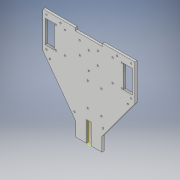
# Autodesk Inventor part: Very real base
Saved by Autodesk Inventor 2019 (Build 230136000, 136)
## iProperties
Created: 2018-08-20
Part Number: Very real base
Material: Generic
Document SubType Name: Modeling
Designer: kalakuntla1297
Density: 1 g/cm^3
Appearance: Default
Author: kalakuntla1297
Autodesk Inventor part; units mm, degrees
ref_plane "YZ Plane" through (0, 0, 0) normal (1, 0, 0) x (0, 1, 0)
ref_plane "XZ Plane" through (0, 0, 0) normal (0, 1, 0) x (-1, 0, 0)
ref_plane "XY Plane" through (0, 0, 0) normal (0, 0, 1) x (1, 0, 0)
sketch "Sketch1" plane through (0, 0, 0) normal (0, 0, 1) x (1, 0, 0)
  line L0 (0, 0) -> (508, 0)
  line L1 (508, 0) -> (508, -185.42)
  line L2 (0, 0) -> (0, -185.42)
  line L3 (254, 0) -> (254, -508)
  line L4 (254, -508) -> (266.7, -508)
  line L5 (254, -508) -> (241.3, -508)
  line L6 (266.7, -508) -> (266.7, -393.7)
  line L7 (241.3, -508) -> (241.3, -393.7)
  line L8 (266.7, -508) -> (326.39, -508)
  line L9 (241.3, -508) -> (181.61, -508)
  line L10 (326.39, -508) -> (326.39, -431.8)
  line L11 (326.39, -431.8) -> (508, -185.42)
  line L12 (241.3, -393.7) -> (266.7, -393.7)
  line L13 (12.7, -22.1996) -> (63.5, -22.1996)
  line L14 (63.5, -22.1996) -> (63.5, -149.1996)
  line L15 (63.5, -149.1996) -> (12.7, -149.1996)
  line L16 (12.7, -149.1996) -> (12.7, -22.1996)
  line L17 (495.3, -22.1996) -> (444.5, -22.1996)
  line L18 (444.5, -22.1996) -> (444.5, -149.1996)
  line L19 (444.5, -149.1996) -> (495.3, -149.1996)
  line L20 (495.3, -149.1996) -> (495.3, -22.1996)
  circle A0 centre (71.374, -24.13) radius 4.064
  circle A1 centre (122.174, -24.13) radius 4.064
  circle A2 centre (71.374, -147.2692) radius 4.064
  circle A3 centre (122.174, -147.2692) radius 4.064
  circle A4 centre (385.826, -147.2692) radius 4.064
  circle A5 centre (436.626, -147.2692) radius 4.064
  circle A6 centre (436.626, -24.13) radius 4.064
  circle A7 centre (385.826, -24.13) radius 4.064
  line L21 (0, -185.42) -> (508, -185.42)
  line L22 (181.61, -508) -> (181.61, -431.8)
  line L23 (181.61, -431.8) -> (0, -185.42)
  dimension "d0" = 508
  dimension "d1" = 185.42
  dimension "d2" = 185.42
  dimension "d3" = 508
  dimension "d4" = 12.7
  dimension "d5" = 12.7
  dimension "d6" = 114.3
  dimension "d7" = 59.69
  dimension "d8" = 59.69
  dimension "d9" = 76.2
  dimension "d10" = 22.1996
  dimension "d11" = 22.1996
  dimension "d12" = 12.7
  dimension "d13" = 12.7
  dimension "d14" = 50.8
  dimension "d15" = 50.8
  dimension "d16" = 149.1996
  dimension "d17" = 149.1996
  dimension "d18" = 8.128
  dimension "d19" = 8.128
  dimension "d20" = 8.128
  dimension "d21" = 8.128
  dimension "d22" = 24.13
  dimension "d23" = 24.13
  dimension "d24" = 147.2692
  dimension "d25" = 147.2692
  dimension "d26" = 7.874
  dimension "d27" = 58.674
  dimension "d28" = 7.874
  dimension "d29" = 58.674
  constraints: 48 end point, 8 centre point, 7 horizontal, 7 vertical, 4 parallel, 4 symmetric about line, 3 perpendicular, 1 midpoint, 1 point on line, 4 other
  measures "d0" distance of L0.start L1.start
  measures "d1" distance of L1.start L11.end
  measures "d2" distance of L0.start L21.start
  measures "d3" distance of L3.start L3.end
  measures "d4" distance of L3.end L6.start
  measures "d5" distance of L3.end L9.start
  measures "d6" distance of L6.start L12.end
  measures "d7" distance of L6.start L10.start
  measures "d8" distance of L9.start L9.end
  measures "d9" distance of L10.start L11.start
  measures "d10" distance between parallel lines of L0 L13
  measures "d11" distance between parallel lines of L0 L17
  measures "d12" distance between parallel lines of L2 L16
  measures "d13" distance between parallel lines of L1 L20
  measures "d14" distance of L14.end L16.start
  measures "d15" distance of L18.end L19.end
  measures "d16" distance between parallel lines of L0 L19
  measures "d17" distance between parallel lines of L0 L15
  measures "d18" diameter of A1
  measures "d19" diameter of A3
  measures "d20" diameter of A2
  measures "d21" diameter of A0
  measures "d22" distance from line of L0 A0.centre
  measures "d23" distance from line of L0 A1.centre
  measures "d24" distance from line of L0 A2.centre
  measures "d25" distance from line of L0 A3.centre
  measures "d26" distance from line of L14 A0.centre
  measures "d27" distance from line of L14 A1.centre
  measures "d28" distance from line of L14 A2.centre
  measures "d29" distance from line of L14 A3.centre
extrude "Extrusion1" add sketch "Sketch1" along normal blind 12.7 contours L0 L3 L21 L2 | L0 L1 L21 L3 | L21 L3 L12 L7 L9 L22 L23 | L21 L11 L10 L8 L6 L12 L3 | L3 L5 L7 L12
sketch "Sketch2" plane through (0, 0, 12.7) normal (0, 0, 1) x (1, 0, 0)
  circle A0 centre (203.2, 9.3133) radius 4.064
  circle A1 centre (304.8, 9.3133) radius 4.064
  circle A2 centre (203.2, -33.02) radius 4.064
  circle A3 centre (304.8, -33.02) radius 4.064
  line L0 (12.7, 15.24) -> (12.7, -185.42)
  line L1 (571.5, -185.42) -> (571.5, 15.24)
  line L2 (508, 0) -> (0, 0) projected
  line L3 (254, 0) -> (177.8, 0)
  line L4 (254, 0) -> (330.2, 0)
  line L5 (177.8, 0) -> (177.8, 31.75)
  line L6 (177.8, 31.75) -> (330.2, 31.75)
  line L7 (330.2, 31.75) -> (330.2, 0)
  point P0 (12.7, -185.42)
  dimension "d33" = 8.128
  dimension "d34" = 8.128
  dimension "d35" = 8.128
  dimension "d36" = 8.128
  dimension "d41" = 190.5
  dimension "d42" = 266.7
  dimension "d43" = 266.7
  dimension "d44" = 190.5
  dimension "d111" = 76.2
  dimension "d112" = 76.2
  dimension "d113" = 31.75
  constraints: 12 end point, 4 centre point, 2 perpendicular, 2 point on line, 1 midpoint, 1 vertical, 3 other
  measures "d33" diameter of A0
  measures "d34" diameter of A1
  measures "d35" diameter of A3
  measures "d36" diameter of A2
  measures "d42" distance from line of L1 A1.centre
  measures "d43" distance from line of L1 A3.centre
  measures "d111" distance of L3.start L3.end
  measures "d112" distance of L4.end L3.start
  measures "d113" distance of L3.end L5.end
extrude "Extrusion3" cut sketch "Sketch2" against normal blind 12.7 contours A2 | A3
extrude "Extrusion4" cut sketch "Sketch1" along normal blind 12.7 contours L12 L6 L4 L3 | L3 L5 L7 L12
sketch "Sketch4" plane through (0, 0, 12.7) normal (0, 0, 1) x (1, 0, 0)
  circle A0 centre (247.65, -336.55) radius 4.064
  circle A1 centre (323.85, -204.47) radius 4.064
  circle A2 centre (323.85, -336.55) radius 4.064
  circle A3 centre (247.65, -204.47) radius 4.064
  line L0 (0, 0) -> (0, -185.42) projected
  line L1 (181.61, -508) -> (241.3, -508) projected
  line L2 (266.7, -508) -> (326.39, -508) projected
  dimension "d51" = 8.128
  dimension "d52" = 8.128
  dimension "d53" = 247.65
  dimension "d54" = 323.85
  dimension "d55" = 247.65
  dimension "d56" = 323.85
  dimension "d57" = 171.45
  dimension "d58" = 171.45
  dimension "d59" = 303.53
  dimension "d60" = 303.53
  dimension "d61" = 8.128
  constraints: 4 centre point, 1 equal radius
  measures "d51" diameter of A1
  measures "d52" diameter of A2
  measures "d53" distance from line of A0.centre L0
  measures "d54" distance from line of A2.centre L0
  measures "d55" distance from line of L0 A3.centre
  measures "d56" distance from line of L0 A1.centre
  measures "d57" distance from line of A0.centre L1
  measures "d58" distance from line of L2 A2.centre
  measures "d59" distance from line of A3.centre L1
  measures "d60" distance from line of L2 A1.centre
  measures "d61" diameter of A0
extrude "Extrusion5" cut sketch "Sketch4" against normal blind 25.4
sketch "Sketch5" plane through (0, 0, 12.7) normal (0, 0, 1) x (1, 0, 0)
  line L0 (0, -185.42) -> (181.61, -431.8) projected
  line L1 (0, -185.42) -> (31.0065, -162.5647)
  circle A0 centre (37.9406, -204.7855) radius 4.1656
  line L2 (181.61, -431.8) -> (181.61, -508) projected
  line L3 (181.61, -431.8) -> (204.5543, -414.8875)
  circle A1 centre (174.3381, -389.8282) radius 4.1656
  point P0 (0, 0)
  dimension "d64" = 90
  dimension "d65" = 8.3312
  dimension "d66" = 19.05
  dimension "d67" = 38.1
  dimension "d68" = 90
  dimension "d69" = 8.3312
  dimension "d70" = 38.1
  dimension "d71" = 19.05
  constraints: 4 end point, 2 centre point
  measures "d64" angle of L0 L1
  measures "d65" diameter of A0
  measures "d66" distance from line of L0 A0.centre
  measures "d67" distance from line of L1 A0.centre
  measures "d68" angle of L0 L3
  measures "d69" diameter of A1
  measures "d70" distance from line of L3 A1.centre
  measures "d71" distance from line of L0 A1.centre
extrude "Extrusion6" cut sketch "Sketch5" against normal blind 25.4
ref_plane "Work Plane1" through (254, -508, 0) normal (1, 0, 0) x (0, 0, -1)
mirror "Mirror1" about plane through (254, -508, 0) normal (1, 0, 0) of "Extrusion6"
sketch "Sketch7" plane through (0, 0, 12.7) normal (0, 0, 1) x (1, 0, 0)
  line L0 (177.8, 0) -> (177.8, 43.18) projected
  line L1 (177.8, 0) -> (0, 0)
  line L2 (0, 0) -> (0, 15.24)
  line L3 (0, 15.24) -> (177.8, 15.24)
  line L4 (177.8, 15.24) -> (177.8, 0)
  dimension "d80" = 15.24
  constraints: 8 end point, 2 parallel, 1 horizontal, 1 perpendicular
  measures "d80" distance of L1.end L2.end
extrude "Extrusion8" add sketch "Sketch7" against normal blind 12.7
mirror "Mirror3" about plane through (254, -508, 0) normal (1, 0, 0) of "Extrusion8"
sketch "Sketch8" plane through (0, 0, 12.7) normal (0, 0, 1) x (1, 0, 0)
  circle A0 centre (96.774, -3.81) radius 4.1656
  line L0 (0, -185.42) -> (0, 15.24) projected
  line L1 (0, 15.24) -> (177.8, 15.24) projected
  point P0 (0, 0)
  dimension "d83" = 8.3312
  dimension "d84" = 96.774
  dimension "d85" = 19.05
  constraints: 1 centre point
  measures "d83" diameter of A0
  measures "d84" distance from line of L0 A0.centre
  measures "d85" distance from line of L1 A0.centre
extrude "Extrusion9" cut sketch "Sketch8" against normal blind 12.7
mirror "Mirror4" about plane through (254, -508, 0) normal (1, 0, 0) of "Extrusion9"
sketch "Sketch9" plane through (0, 0, 12.7) normal (0, 0, 1) x (1, 0, 0)
  circle A0 centre (19.05, -1.397) radius 4.1656
  line L0 (0, -185.42) -> (0, 15.24) projected
  line L1 (0, 15.24) -> (177.8, 15.24) projected
  point P0 (0, 0)
  dimension "d88" = 8.3312
  dimension "d89" = 19.05
  dimension "d90" = 16.637
  constraints: 1 centre point
  measures "d88" diameter of A0
  measures "d89" distance from line of L0 A0.centre
  measures "d90" distance from line of L1 A0.centre
extrude "Extrusion10" cut sketch "Sketch9" against normal blind 12.7
mirror "Mirror5" about plane through (254, -508, 0) normal (1, 0, 0) of "Extrusion10"
sketch "Sketch10" plane through (0, 0, 12.7) normal (0, 0, 1) x (1, 0, 0)
  line L0 (0, -185.42) -> (181.61, -431.8) projected
  line L1 (0, -185.42) -> (68.7917, -185.42)
  circle A0 centre (19.05, -168.783) radius 4.1656
  line L2 (0, -185.42) -> (0, 15.24) projected
  point P0 (0, 0)
  dimension "d93" = 8.3312
  dimension "d94" = 19.05
  dimension "d95" = 16.637
  constraints: 2 end point, 1 centre point, 1 horizontal
  measures "d93" diameter of A0
  measures "d94" distance from line of L2 A0.centre
  measures "d95" distance from line of L1 A0.centre
extrude "Extrusion11" cut sketch "Sketch10" against normal blind 12.7
mirror "Mirror6" about plane through (254, -508, 0) normal (1, 0, 0) of "Extrusion11"
sketch "Sketch11" plane through (0, 0, 12.7) normal (0, 0, 1) x (1, 0, 0)
  circle A0 centre (254, -55.7555) radius 4.064
  circle A1 centre (203.2, -33.02) radius 4.064 projected
  circle A2 centre (254, -154.1805) radius 4.064
  circle A3 centre (303.2125, -104.9553) radius 4.064
  circle A4 centre (204.7875, -104.9553) radius 4.064
  circle A5 centre (304.8, -33.02) radius 4.064 projected
  point P0 (0, 0)
  dimension "d99" = 8.128
  dimension "d100" = 50.8
  dimension "d101" = 8.128
  dimension "d102" = 98.425
  dimension "d103" = 8.128
  dimension "d104" = 8.128
  dimension "d105" = 98.425
  dimension "d106" = 1.5875
  dimension "d107" = 49.2252
  constraints: 4 centre point
  measures "d99" diameter of A0
  measures "d100" horizontal distance of A1.centre A0.centre
  measures "d101" diameter of A2
  measures "d102" distance between centres of A0 A2
  measures "d103" diameter of A4
  measures "d104" diameter of A3
  measures "d105" distance of A3.centre A4.centre
  measures "d106" horizontal distance of A5.centre A3.centre
  measures "d107" vertical distance of A4.centre A2.centre
extrude "Extrusion12" cut sketch "Sketch11" against normal blind 25.4 contours A0 | A2 | A3 | A4
body "Solid1"
